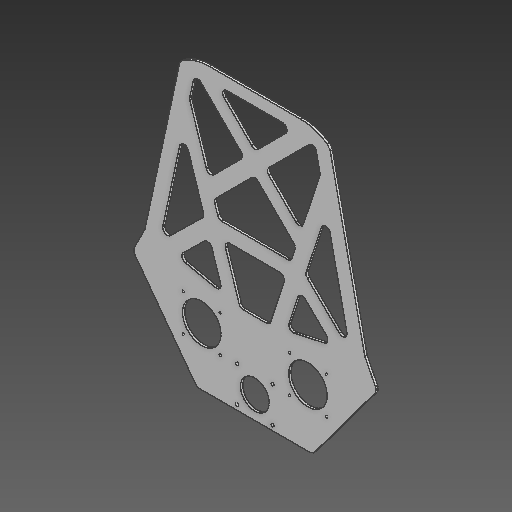
# Autodesk Inventor part: ChestFrontPanel
Saved by Autodesk Inventor 2025.2 (Build 292293000, 293)
## iProperties
Created: 2025-09-23
Part Number: ChestFrontPanel
Material: Generic
Document SubType Name: Sheet Metal
Designer: valer
Density: 1 g/cm^3
Sheet Metal Rule: Default_mm
Appearance: Default
Author: valer
Autodesk Inventor part; units mm, degrees
ref_plane "YZ Plane" through (0, 0, 0) normal (1, 0, 0) x (0, 1, 0)
ref_plane "XZ Plane" through (0, 0, 0) normal (0, 1, 0) x (-1, 0, 0)
ref_plane "XY Plane" through (0, 0, 0) normal (0, 0, 1) x (1, 0, 0)
sketch "Base" plane through (0, 0, 0) normal (0, 0, 1) x (1, 0, 0)
  line L0 (-341.7653, 0) -> (341.7653, 0) construction
  line L1 (0, -75.5138) -> (0, 453.0828) construction
  line L2 (183.676, 264.154) -> (223.6199, 230.6371) construction
  arc A0 (180.154, 267.676) -> (183.676, 264.154) centre (202.0437, 286.0437) ccw construction
  line L3 (105.6111, 356.5128) -> (180.154, 267.676) construction
  arc A1 (105.6111, 356.5128) -> (69.1282, 373.525) centre (69.1282, 325.9) ccw construction
  line L4 (-69.1282, 373.525) -> (69.1282, 373.525) construction
  arc A2 (231.2425, 165.7605) -> (223.6199, 230.6371) centre (193.0071, 194.1542) ccw construction
  line L5 (231.2425, 165.7605) -> (183.8243, 101.9065) construction
  line L6 (0, 373.525) -> (69.1282, 373.525) construction
  line L7 (183.8243, 101.9065) -> (108.1482, 0) construction
  line L8 (-183.676, 264.154) -> (-223.6199, 230.6371) construction
  arc A3 (-183.676, 264.154) -> (-180.154, 267.676) centre (-202.0437, 286.0437) ccw construction
  line L9 (-105.6111, 356.5128) -> (-180.154, 267.676) construction
  arc A4 (-69.1282, 373.525) -> (-105.6111, 356.5128) centre (-69.1282, 325.9) ccw construction
  arc A5 (-223.6199, 230.6371) -> (-231.2425, 165.7605) centre (-193.0071, 194.1542) ccw construction
  line L10 (-231.2425, 165.7605) -> (-183.8243, 101.9065) construction
  line L11 (0, 373.525) -> (-69.1282, 373.525) construction
  line L12 (-183.8243, 101.9065) -> (-108.1482, 0) construction
  line L13 (108.1482, 0) -> (-108.1482, 0)
  line L14 (-108.1482, 0) -> (-186.1215, 105)
  line L15 (-186.1215, 105) -> (186.1215, 105)
  line L16 (186.1215, 105) -> (108.1482, 0)
  point P0 (0, 105)
extrude "Plate1" add sketch "Base" along normal blind 3
chamfer "SideChamferFeature" distance 40 angle 45 2 edges at (-186.1215, 105, 1.5) (186.1215, 105, 1.5)
fillet "OutsideFillets1Feature" radius 8 4 edges at (108.1482, 0, 1.5) (162.2738, 72.8863, 1.5) (-108.1482, 0, 1.5) (-162.2738, 72.8863, 1.5)
sketch "Mount" plane through (0, 0, 0) normal (0, 0, -1) x (-1, 0, 0)
  line L0 (-146.1215, 105) -> (146.1215, 105)
  line L1 (-146.1215, 105) -> (-89.2554, 369.0629)
  line L2 (0, -75.5138) -> (0, 453.0828) construction
  line L3 (-89.2554, 369.0629) -> (0, 369.0629)
  arc A0 (-69.1282, 373.525) -> (-105.6111, 356.5128) centre (-69.1282, 325.9) ccw construction
  line L4 (146.1215, 105) -> (89.2554, 369.0629)
  line L5 (89.2554, 369.0629) -> (0, 369.0629)
  point P0 (0, 0)
sheet face with bend "MountFeature" sketch "Mount" thickness 3 toward (0, 0, 1) bend radius 3
bend "Bend1"
fillet "TopFilletsFeature" radius 8 2 edges at (89.2554, 369.0629, 1.5) (-89.2554, 369.0629, 1.5)
sketch "ExternalHoles" plane through (0, 0, 0) normal (0, 0, -1) x (-1, 0, 0)
  circle A0 centre (20, 67) radius 2.7 projected
  circle A1 centre (20, 85) radius 2.7 projected
  circle A2 centre (-20, 67) radius 2.7 projected
  circle A3 centre (-20, 85) radius 2.7 projected
  circle A4 centre (95.1, 10) radius 1.5 projected
  circle A5 centre (70.6, 34.5) radius 25.5 projected
  circle A6 centre (95.1, 59) radius 1.5 projected
  circle A7 centre (46.1, 59) radius 1.5 projected
  circle A8 centre (46.1, 10) radius 1.5 projected
  circle A9 centre (-70.6, 34.5) radius 25.5 projected
  circle A10 centre (-95.1, 10) radius 1.5 projected
  circle A11 centre (-46.1, 10) radius 1.5 projected
  circle A12 centre (-95.1, 59) radius 1.5 projected
  circle A13 centre (-46.1, 59) radius 1.5 projected
  point P0 (0, 0)
extrude "MeterMountHolesFeature" cut sketch "ExternalHoles" against normal blind 3 contours A4 | A5 | A6 | A7 | A8 | A9 | A10 | A11 | A12 | A13
sketch "Profile" plane through (0, 0, 0) normal (0, 0, -1) x (-1, 0, 0)
  line L0 (-146.1215, 105) -> (-160.0581, 77.2916) projected
  line L1 (-153.0898, 91.1458) -> (153.0898, 91.1458)
  line L2 (160.0581, 77.2916) -> (146.1215, 105) projected
  line L3 (-90.6155, 362.7471) -> (-146.1215, 105) projected
  line L4 (-107.609, 283.8364) -> (-45, 91.1458)
  line L5 (0, -74.0889) -> (0, 444.5336) construction
  line L6 (107.609, 283.8364) -> (45, 91.1458)
  line L7 (146.1215, 105) -> (90.6155, 362.7471) projected
  arc A0 (-82.7948, 369.0629) -> (-90.6155, 362.7471) centre (-82.7948, 361.0629) ccw projected
  line L8 (82.7948, 369.0629) -> (-82.7948, 369.0629) projected
  arc A1 (90.6155, 362.7471) -> (82.7948, 369.0629) centre (82.7948, 361.0629) ccw projected
  line L9 (69.1282, 339.3119) -> (-69.1282, 339.3119) construction
  line L10 (-95.6623, 339.3119) -> (95.6623, 339.3119)
  point P0 (0, 0)
  dimension "d62" = 72
  dimension "d63" = 90
  constraints: 10 end point, 4 point on line, 2 horizontal, 2 midpoint, 2 symmetric about line, 1 collinear, 2 other
  measures "d62" angle of L1 L4
  measures "d63" distance of L6.end L4.end
extrude "ProfileFeature" cut sketch "Profile" against normal blind 3 contours L3 A0 L8 A1 L7 L10
fillet "ProfileFilletFeature" radius 8 2 edges at (95.6623, 339.3119, 1.5) (-95.6623, 339.3119, 1.5)
sketch "MountHoles" plane through (0, 0, 0) normal (0, 0, -1) x (-1, 0, 0)
  line L0 (0, -67.8624) -> (0, 407.1743) construction
  circle A0 centre (-148, 73.6458) radius 3
  line L1 (-148, 73.6458) -> (0, 73.6458) construction
  circle A1 centre (0, 73.6458) radius 3 construction
  circle A2 centre (-74, 73.6458) radius 3
  line L2 (69.1282, 321.9129) -> (-69.1282, 321.9129) construction
  line L3 (-69.1282, 321.9129) -> (-69.1282, 339.3119) construction
  line L4 (89.2017, 339.3119) -> (-89.2017, 339.3119) projected
  line L5 (-97.0224, 332.9961) -> (-146.1215, 105) projected
  line L6 (-97.5357, 330.6124) -> (0, 330.6124) construction
  circle A3 centre (-88.8409, 330.6124) radius 3
  circle A4 centre (0, 330.6124) radius 3
  circle A5 centre (-48.7679, 330.6124) radius 3
  circle A6 centre (148, 73.6458) radius 3
  circle A7 centre (74, 73.6458) radius 3
  circle A8 centre (88.8409, 330.6124) radius 3
  circle A9 centre (48.7679, 330.6124) radius 3
  line L7 (104.1244, 0) -> (-104.1244, 0) projected
  point P0 (0, 0)
  point P1 (-107.1553, 285.9432)
  point P2 (-69.1282, 330.6124)
  dimension "d70" = 6
  dimension "d72" = 6
  dimension "d73" = 6
  dimension "d74" = 6
  dimension "d75" = 8.5
  dimension "d76" = 6
  dimension "d77" = 6
  dimension "d98" = 73.6458
  dimension "d104" = 74
  dimension "d105" = 74
  constraints: 10 centre point, 8 end point, 6 point on line, 4 symmetric about line, 3 midpoint, 2 coincident, 2 perpendicular, 1 horizontal, 1 vertical, 6 other
  measures "d70" diameter of A0
  measures "d72" diameter of A1
  measures "d73" diameter of A2
  measures "d74" diameter of A3
  measures "d75" distance from line of L5 A3.centre
  measures "d76" diameter of A4
  measures "d77" diameter of A5
  measures "d98" distance between parallel lines of L7 L1
  measures "d104" distance from line of L0 A2.centre
  measures "d105" distance of L1.start A2.centre
cut "MountHolesFeature" [suppressed]
sketch "Holes" plane through (0, 0, 0) normal (0, 0, -1) x (-1, 0, 0)
  line L0 (-86.923, 284.8928) -> (-79.5108, 319.3119)
  line L1 (-79.5108, 319.3119) -> (-14.1421, 253.9432)
  line L2 (-14.1421, 253.9432) -> (-61.4844, 206.601)
  line L3 (-61.4844, 206.601) -> (-86.923, 284.8928)
  line L4 (-54.548, 185.2531) -> (0, 239.8011)
  line L5 (0, 239.8011) -> (54.548, 185.2531)
  line L6 (54.548, 185.2531) -> (-54.548, 185.2531) construction
  line L7 (0, -67.8624) -> (0, 407.1743) construction
  line L8 (86.923, 284.8928) -> (79.5108, 319.3119)
  line L9 (79.5108, 319.3119) -> (14.1421, 253.9432)
  line L10 (14.1421, 253.9432) -> (61.4844, 206.601)
  line L11 (61.4844, 206.601) -> (86.923, 284.8928)
  line L12 (-51.2265, 319.3119) -> (51.2265, 319.3119)
  line L13 (51.2265, 319.3119) -> (0, 268.0854)
  line L14 (-51.2265, 319.3119) -> (0, 268.0854)
  line L15 (-79.5108, 319.3119) -> (-51.2265, 319.3119) construction
  line L16 (51.2265, 319.3119) -> (79.5108, 319.3119) construction
  line L17 (89.2017, 339.3119) -> (-89.2017, 339.3119) projected
  line L18 (-97.0224, 332.9961) -> (-146.1215, 105) projected
  line L19 (-61.4844, 206.601) -> (-54.548, 185.2531) construction
  line L20 (-48.0497, 165.2531) -> (48.0497, 165.2531)
  line L21 (-54.548, 185.2531) -> (-48.0497, 165.2531)
  line L22 (-95.3052, 245.9693) -> (-67.0708, 159.0727)
  line L23 (-67.0708, 159.0727) -> (-126.5697, 100.7895)
  line L24 (-126.5697, 100.7895) -> (-95.3052, 245.9693)
  line L25 (-67.0708, 159.0727) -> (-48.0497, 165.2531) construction
  line L26 (-146.1215, 105) -> (-126.5697, 100.7895) construction
  line L27 (54.548, 185.2531) -> (48.0497, 165.2531)
  line L28 (95.3052, 245.9693) -> (67.0708, 159.0727)
  line L29 (67.0708, 159.0727) -> (126.5697, 100.7895)
  line L30 (126.5697, 100.7895) -> (95.3052, 245.9693)
  line L31 (67.0708, 159.0727) -> (48.0497, 165.2531) construction
  line L32 (-103.1398, 95.7439) -> (-60.1704, 137.8354)
  line L33 (-60.1704, 137.8354) -> (-42.2322, 82.6274)
  line L34 (-42.2322, 82.6274) -> (-103.1398, 95.7439)
  line L35 (0, 145.2531) -> (-41.5513, 145.2531)
  line L36 (-41.5513, 145.2531) -> (-19.6208, 77.758)
  line L37 (-19.6208, 77.758) -> (0, 77.758)
  line L38 (-126.5697, 100.7895) -> (-19.6208, 77.758) construction
  line L39 (103.1398, 95.7439) -> (60.1704, 137.8354)
  line L40 (60.1704, 137.8354) -> (42.2322, 82.6274)
  line L41 (42.2322, 82.6274) -> (103.1398, 95.7439)
  line L42 (0, 145.2531) -> (41.5513, 145.2531)
  line L43 (41.5513, 145.2531) -> (19.6208, 77.758)
  line L44 (19.6208, 77.758) -> (0, 77.758)
  line L45 (126.5697, 100.7895) -> (19.6208, 77.758) construction
  point P0 (0, 0)
  point P1 (0, 165.2531)
  dimension "d80" = 20
  dimension "d81" = 20
  dimension "d82" = 20
  dimension "d84" = 20
  dimension "d85" = 20
  dimension "d99" = 30.153
  dimension "d100" = 132.7109
  dimension "d101" = 20
  dimension "d102" = 20
  dimension "d103" = 20
  constraints: 86 end point, 12 symmetric about line, 9 parallel, 8 collinear, 6 point on line, 5 perpendicular, 4 horizontal, 1 midpoint
  measures "d80" distance between parallel lines of L1 L14
  measures "d81" distance between parallel lines of L17 L12
  measures "d82" distance between parallel lines of L0 L18
  measures "d84" distance between parallel lines of L4 L2
  measures "d85" distance between parallel lines of L20 L6
  measures "d99" angle of L18 L3
  measures "d100" distance from line of L17 L2.end
  measures "d101" distance between parallel lines of L3 L22
  measures "d102" distance between parallel lines of L32 L23
  measures "d103" distance between parallel lines of L20 L35
extrude "HolesFeature" cut sketch "Holes" against normal through all
fillet "InsideFilletsFeature" radius 6 32 edges at (79.5108, 319.3119, 1.5) (86.923, 284.8928, 1.5) (61.4844, 206.601, 1.5) (14.1421, 253.9432, 1.5) (51.2265, 319.3119, 1.5) (-51.2265, 319.3119, 1.5) (0, 268.0854, 1.5) (-79.5108, 319.3119, 1.5) (-14.1421, 253.9432, 1.5) (-86.923, 284.8928, 1.5) (-61.4844, 206.601, 1.5) (0, 239.8011, 1.5) (-54.548, 185.2531, 1.5) (54.548, 185.2531, 1.5) (48.0497, 165.2531, 1.5) (-48.0497, 165.2531, 1.5) (95.3052, 245.9693, 1.5) (126.5697, 100.7895, 1.5) (67.0708, 159.0727, 1.5) (60.1704, 137.8354, 1.5) (103.1398, 95.7439, 1.5) (42.2322, 82.6274, 1.5) (41.5513, 145.2531, 1.5) (19.6208, 77.758, 1.5) (-41.5513, 145.2531, 1.5) (-19.6208, 77.758, 1.5) (-60.1704, 137.8354, 1.5) (-42.2322, 82.6274, 1.5) (-103.1398, 95.7439, 1.5) (-95.3052, 245.9693, 1.5) (-67.0708, 159.0727, 1.5) (-126.5697, 100.7895, 1.5)
sketch "BottomExtension" plane through (0, 0, 0) normal (0, 0, -1) x (-1, 0, 0)
  line L0 (-159.3339, 68.9274) -> (-110.5471, 3.2305)
  line L1 (-110.5471, 3.2305) -> (-76.9589, -42)
  line L2 (-76.9589, -42) -> (0, -42)
  line L3 (0, -42) -> (0, 0) construction
  line L4 (104.1244, 0) -> (-104.1244, 0)
  arc A0 (-110.5471, 3.2305) -> (-104.1244, 0) centre (-104.1244, 8) ccw
  line L5 (110.5471, 3.2305) -> (76.9589, -42)
  line L6 (76.9589, -42) -> (0, -42)
  arc A1 (104.1244, 0) -> (110.5471, 3.2305) centre (104.1244, 8) ccw
  dimension "d89" = 42
  measures "d89" distance between parallel lines of L2 L4
sheet face with bend "BottomExtensionFeature" sketch "BottomExtension" thickness 3 toward (0, 0, 1) bend radius 3
bend "Bend2"
fillet "AdditionalFilletsFeature" radius 8 2 edges at (76.9589, -42, 1.5) (-76.9589, -42, 1.5)
sketch "NeckGearboxMountHoles" plane through (0, 0, 0) normal (0, 0, -1) x (-1, 0, 0)
  circle A0 centre (0, -12) radius 19.05 projected
  circle A1 centre (-23.57, -35.57) radius 2 projected
  circle A2 centre (23.57, -35.57) radius 2 projected
  circle A3 centre (-23.57, 11.57) radius 2 projected
  circle A4 centre (23.57, 11.57) radius 2 projected
  point P0 (0, 0)
extrude "NeckGearboxMountHolesFeature" cut sketch "NeckGearboxMountHoles" against normal through all
sketch "Sketch16" plane through (0, 0, 3) normal (0, 0, 1) x (1, 0, 0)
  line L0 (-146.1215, 105) -> (-97.0224, 332.9961) projected
  arc A0 (-60.3986, 335.3119) -> (-99.4434, 321.7538) centre (-60.3986, 272.3119) ccw
  line L1 (-60.3986, 335.3119) -> (0, 335.3119)
  line L2 (89.2017, 339.3119) -> (-89.2017, 339.3119) projected
  line L3 (0, -118.5387) -> (0, 417.2324) construction
  arc A1 (99.4434, 321.7538) -> (60.3986, 335.3119) centre (60.3986, 272.3119) ccw
  line L4 (60.3986, 335.3119) -> (0, 335.3119)
  arc A2 (-89.2017, 339.3119) -> (-97.0224, 332.9961) centre (-89.2017, 331.3119) ccw projected
  arc A3 (97.0224, 332.9961) -> (89.2017, 339.3119) centre (89.2017, 331.3119) ccw projected
  line L5 (97.0224, 332.9961) -> (146.1215, 105) projected
  point P0 (0, 0)
  dimension "d106" = 4
  dimension "d107" = 11.5
  dimension "d108" = 63
  constraints: 4 end point, 4 point on circle, 3 symmetric about line, 2 centre point, 1 horizontal, 1 point on line, 1 tangent, 1 other
  measures "d106" distance between parallel lines of L2 L1
  measures "d107" distance of L0.end A0.end
  measures "d108" radius of A0
extrude "Cut10" cut sketch "Sketch16" against normal blind 3
fillet "Fillet7" radius 10 2 edges at (-99.4434, 321.7538, 1.5) (99.4434, 321.7538, 1.5)
equation "\"d0\" = Thickness"
equation "\"d17\" = BendRadius"
equation "\"d18\" = BendReliefWidth"
equation "\"d20\" = MinimumRemnant"
equation "\"d19\" = BendReliefDepth"
equation "\"d21\" = TransitionRadius"
equation "\"BendRadius\" = Thickness"
equation "\"BendReliefWidth\" = Thickness"
equation "\"BendReliefDepth\" = 0.5 * Thickness"
equation "\"CornerReliefSize\" = 4 * Thickness"
equation "\"MinimumRemnant\" = 2 * Thickness"
equation "\"TransitionRadius\" = BendRadius"
equation "\"JacobiRadiusSize\" = BendRadius"
equation "\"GapSize\" = Thickness"
equation "\"Thickness\" = 3"
body "Solid1"
